BGCCornerHolder (Autodesk Fusion 360 design; units mm, degrees)
Autodesk Fusion 360 part; units mm, degrees
sketch "Sketch1" plane through (0, 0, 0) normal (0, 1, 0) x (1, 0, 0)
  circle A0 centre (0, 0) radius 3
  circle A1 centre (0, 0) radius 5
  line L0 (5, -1) -> (7, -1)
  line L1 (7, -1) -> (7, 51)
  line L2 (7, 51) -> (5, 51)
  line L3 (5, 51) -> (5, -1)
  line L4 (5, 25) -> (0, 25) construction
  line L5 (0, 25) -> (0, 0) construction
  line L6 (0, 0) -> (0, -10) construction
  line L7 (0, 5) -> (10, 5) construction
  line L8 (10, 5) -> (10, 0)
  arc A2 (0, -10) -> (10, 0) centre (0, 0) ccw
  line L9 (10, 5) -> (7, 5)
  line L10 (5, 5) -> (0, 5)
  line L11 (-5, 5) -> (0, 5)
  line L12 (-5, 51) -> (-5, -1)
  line L13 (-5, -1) -> (-7, -1)
  line L14 (-7, -1) -> (-7, 51)
  line L15 (-10, 5) -> (-7, 5)
  arc A3 (-10, 0) -> (0, -10) centre (0, 0) ccw
  line L16 (-10, 5) -> (-10, 0)
  dimension "d1" = 6
  dimension "d2" = 10
  dimension "d3" = 2
  dimension "d4" = 52
  dimension "d5" = 25
  dimension "d6" = 10
  dimension "d7" = 10
  dimension "d8" = 5
  constraint coincident A0.centre A1.centre
  constraint horizontal L0
  constraint vertical L1
  constraint horizontal L2
  constraint vertical L3
  constraint coincident L3 L4.start
  constraint perpendicular L3 L4
  constraint perpendicular L4 L5
  constraint midpoint L3 L4.start
  constraint tangent A1 L3
  constraint parallel L5 L6
  constraint coincident A1 L7.start
  constraint coincident L5 L7.start
  constraint perpendicular L1 L7
  constraint perpendicular L7 L8
  constraint tangent L8 A2
  constraint coincident L6 A2.start
  constraint coincident L6.end A2.start
  constraint coincident L1 L9.end
  constraint coincident L7 L9.end
  constraint midpoint L7 L10.start
  constraint symmetric L0.start L5 L12.end
  constraint symmetric L0.end L5 L13.end
  constraint symmetric L1.end L5 L14.end
  constraint symmetric L2.end L5 L12.start
  constraint symmetric L5 L7.start L10.end
  constraint symmetric L5 L7.end L15.start
  constraint symmetric L5 L8.end A3.start
  constraint symmetric L5 L6.end A2.start
  constraint symmetric L5 A2 A3
  constraint symmetric L5 L9.end L15.end
  constraint symmetric L5 L10.start L11.start
  measures "d1" diameter of A0
  measures "d2" diameter of A1
  measures "d3" distance of L0.start L0.end
  measures "d4" distance of L0.start L2.end
  measures "d5" distance of L4.end A0.centre
  measures "d6" distance of L7.start L7.end
  measures "d7" distance of A0.centre L6.end
  measures "d8" distance of L7.end L8.end
extrude "Extrude1" add sketch "Sketch1" along normal blind 5 contours A1 | A1 L0 L1 L3 L8 A2 L9 L12 L13 L14 L15 A3 L16 | A1 L3 L10 | A1 L11 L12
sketch "Sketch2" plane through (0, 0, 0) normal (0, -1, 0) x (1, 0, 0)
  circle A0 centre (0, 0) radius 3
  line L0 (-5, 1) -> (-5, -5)
  line L1 (-5, -5) -> (5, -5)
  line L2 (5, -5) -> (5, 1)
  line L3 (5, 1) -> (7, 1)
  line L4 (7, 1) -> (7, -5)
  line L5 (7, -5) -> (10, -5)
  line L6 (10, -5) -> (10, 0)
  arc A1 (10, 0) -> (-10, 0) centre (0, 0) ccw
  line L7 (-10, 0) -> (-10, -5)
  line L8 (-10, -5) -> (-7, -5)
  line L9 (-7, -5) -> (-7, 1)
  line L10 (-7, 1) -> (-5, 1)
  line L11 (10, -5) -> (-10, -5)
  constraint coincident L5.end L6.start
  constraint coincident L7.end L8.start
extrude "Extrude2" add sketch "Sketch2" along normal blind 5
